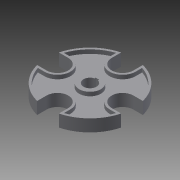
# Autodesk Inventor part: 基准图-装填桶
Saved by Autodesk Inventor 2015 (Build 190159000, 159)
## iProperties
Created: 2017-05-03
Part Number: 基准图-装填桶
Material: 常规
Document SubType Name: Modeling
Designer: Administrator
Density: 1 g/cm^3
Appearance: 默认
Author: Administrator
Autodesk Inventor part; units mm, degrees
ref_plane "YZ Plane" through (0, 0, 0) normal (1, 0, 0) x (0, 1, 0)
ref_plane "XZ Plane" through (0, 0, 0) normal (0, 1, 0) x (-1, 0, 0)
ref_plane "XY Plane" through (0, 0, 0) normal (0, 0, 1) x (1, 0, 0)
sketch "草图1" plane through (0, 0, 0) normal (0, 0, 1) x (1, 0, 0)
  arc A0 (25, -75) -> (-25, -75) centre (0, -75) ccw
  line L0 (-25, -75) -> (-25, -96.8246)
  line L1 (25, -75) -> (25, -96.8246)
  line L2 (0, 0) -> (9.4022, 0)
  line L3 (0, 0) -> (0, -9.3611)
  arc A1 (75, 25) -> (75, -25) centre (75, 0) ccw
  line L4 (75, -25) -> (96.8246, -25)
  line L5 (75, 25) -> (96.8246, 25)
  arc A2 (-25, 75) -> (25, 75) centre (0, 75) ccw
  line L6 (25, 75) -> (25, 96.8246)
  line L7 (-25, 75) -> (-25, 96.8246)
  arc A3 (-75, -25) -> (-75, 25) centre (-75, 0) ccw
  line L8 (-75, 25) -> (-96.8246, 25)
  line L9 (-75, -25) -> (-96.8246, -25)
  arc A4 (-25, 96.8246) -> (-96.8246, 25) centre (0, 0) ccw
  arc A5 (96.8246, 25) -> (25, 96.8246) centre (0, 0) ccw
  arc A6 (-96.8246, -25) -> (-25, -96.8246) centre (0, 0) ccw
  arc A7 (25, -96.8246) -> (96.8246, -25) centre (0, 0) ccw
  dimension "d0" = 50
  dimension "d2" = 9.4022
  dimension "d3" = 9.3611
  dimension "d6" = 360
  dimension "d12" = 100
  constraints: 20 end point, 16 point on circle, 8 centre point, 3 tangent, 2 vertical, 1 coincident, 1 horizontal, 1 parallel, 1 point on line, 33 other
  measures "d0" diameter of A0
  measures "d2" distance of L2.start L2.end
  measures "d3" distance of L2.start L3.end
  measures "d12" radius of A5
extrude "拉伸1" add sketch "草图1" along normal blind 28
sketch "草图2" plane through (0, 0, 28) normal (0, 0, 1) x (1, 0, 0)
  circle A0 centre (0, 0) radius 25
  arc A1 (30, -75) -> (-30, -75) centre (0, -75) ccw
  arc A2 (25, -75) -> (-25, -75) centre (0, -75) ccw projected
  line L0 (30, -75) -> (30, -90.1388)
  line L1 (-30, -75) -> (-30, -90.1388)
  arc A3 (75, 30) -> (75, -30) centre (75, 0) ccw
  line L2 (75, 30) -> (90.1388, 30)
  line L3 (75, -30) -> (90.1388, -30)
  arc A4 (-30, 75) -> (30, 75) centre (0, 75) ccw
  line L4 (-30, 75) -> (-30, 90.1388)
  line L5 (30, 75) -> (30, 90.1388)
  arc A5 (-75, -30) -> (-75, 30) centre (-75, 0) ccw
  line L6 (-75, -30) -> (-90.1388, -30)
  line L7 (-75, 30) -> (-90.1388, 30)
  arc A6 (-90.1388, -30) -> (-30, -90.1388) centre (0, 0) ccw
  arc A7 (-30, 90.1388) -> (-90.1388, 30) centre (0, 0) ccw
  arc A8 (30, -90.1388) -> (90.1388, -30) centre (0, 0) ccw
  arc A9 (90.1388, 30) -> (30, 90.1388) centre (0, 0) ccw
  dimension "d15" = 50
  dimension "d17" = 5
  dimension "d20" = 360
  dimension "d22" = 95
  constraints: 16 end point, 16 point on circle, 9 centre point, 2 coincident, 2 tangent, 1 concentric, 1 parallel, 1 vertical, 33 other
  measures "d15" diameter of A0
  measures "d17" radial gap between concentric circles of A2 A1
  measures "d22" radius of A9
extrude "拉伸2" cut sketch "草图2" against normal blind 9
pattern_linear "矩形阵列1" count 2 spacing 19 along (0, 0, -1) of "拉伸2"
sketch "草图3" plane through (0, 0, 28) normal (0, 0, 1) x (1, 0, 0)
  circle A0 centre (0, 0) radius 15
  line L0 (-4, 14.4568) -> (4, 14.4568)
  line L1 (4, 14.4568) -> (4, 17.2)
  line L2 (4, 17.2) -> (-4, 17.2)
  line L3 (-4, 17.2) -> (-4, 14.4568)
  dimension "d28" = 30
  dimension "d29" = 17.2
  dimension "d30" = 8
  constraints: 8 end point, 2 parallel, 2 point on circle, 1 centre point, 1 coincident, 1 horizontal, 1 perpendicular
  measures "d28" diameter of A0
  measures "d29" distance from line of point (0, 0) L2
  measures "d30" distance of L0.start L0.end
extrude "拉伸3" cut sketch "草图3" against normal blind 28
